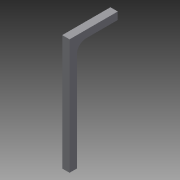
# Autodesk Inventor part: allen key
Saved by Autodesk Inventor 2015 (Build 190159000, 159)
## iProperties
Created: 2014-11-04
Part Number: allen key
Material: Generic
Document SubType Name: Modeling
Designer: jesse
Density: 1 g/cm^3
Appearance: Default
Author: jesse
Autodesk Inventor part; units mm, degrees
ref_plane "YZ Plane" through (0, 0, 0) normal (1, 0, 0) x (0, 1, 0)
ref_plane "XZ Plane" through (0, 0, 0) normal (0, 1, 0) x (-1, 0, 0)
ref_plane "XY Plane" through (0, 0, 0) normal (0, 0, 1) x (1, 0, 0)
sketch "Sketch1" plane through (0, 0, 0) normal (1, 0, 0) x (0, 1, 0)
  line L0 (0, 0) -> (39.8649, 0)
  line L1 (39.8649, 0) -> (39.8649, -16.6447)
  line L2 (39.8649, -16.6447) -> (37.3249, -16.6447)
  line L3 (37.3249, -16.6447) -> (37.3249, -5.715)
  line L4 (34.1499, -2.54) -> (0, -2.54)
  line L5 (0, -2.54) -> (0, 0)
  arc A0 (37.3249, -5.715) -> (34.1499, -2.54) centre (34.1499, -5.715) ccw
  dimension "d0" = 2.54
  dimension "d1" = 3.175
  constraints: 12 end point, 6 perpendicular, 2 point on circle, 2 tangent, 1 centre point, 1 horizontal
  measures "d0" distance of L1.end L2.end
  measures "d1" radius of A0
extrude "Extrusion1" add sketch "Sketch1" along normal blind 2.54
body "Solid1"
